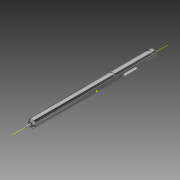
# Autodesk Inventor part: Motor shaft
Saved by Autodesk Inventor 2015 (Build 190141000, 141)
## iProperties
Created: 2008-06-08
Part Number: Motor shaft
Document SubType Name: Modeling
Designer: tangg
Density: 7.84 g/cm^3
Mass: 17.005 g
Surface Area: 63.6795 cm^2
Volume: 17.005 cm^3
Material: Steel, High Strength Low Alloy
Appearance: Steel - Polished
Author: tangg
Autodesk Inventor part; units mm, degrees
ref_plane "XZ Plane" through (0, 0, 0) normal (0, 1, 0) x (-1, 0, 0)
sketch "Sketch1" plane through (0, 0, 0) normal (0, 0, 1) x (1, 0, 0)
  circle A0 centre (0, 0) radius 5
  dimension "d0" = 10
  constraints: 1 centre point, 1 coincident
  measures "d0" diameter of A0
extrude "Extrusion1" add sketch "Sketch1" along normal mid plane 152.4
ref_plane "Work Plane4" through (0, 0, 0) normal (0, 0, 1) x (1, 0, 0)
ref_plane "Work Plane5" through (0, 0, -2) normal (0, 0, 1) x (1, 0, 0)
ref_plane "Work Plane6" through (5, 0, 0) normal (1, 0, 0) x (0, 1, 0)
sketch "Sketch6" plane through (5, 0, 0) normal (1, 0, 0) x (0, 1, 0)
  point P0 (0, 0)
sketch "Sketch7" plane through (5, 0, 0) normal (1, 0, 0) x (0, 1, 0)
  line L0 (0, 106.68) -> (0, -106.68) projected
  line L1 (-1.5, -49.2154) -> (-1.5272, -34.9251)
  line L2 (1.4728, -34.9193) -> (1.5, -49.2096)
  arc A0 (-1.5, -49.2154) -> (1.5, -49.2096) centre (0, -49.2125) ccw
  arc A1 (1.4728, -34.9193) -> (-1.5272, -34.9251) centre (-0.0272, -34.9222) ccw
  line L3 (-1.5, -49.2154) -> (1.5, -49.2096) construction
  line L4 (-1.5272, -34.9251) -> (1.4728, -34.9193) construction
  point P0 (0, 0)
  dimension "d28" = 3
  constraints: 8 end point, 5 point on circle, 3 tangent, 2 centre point, 2 midpoint, 1 coincident, 1 point on line
  measures "d28" distance between parallel lines of L1 L2
extrude "Extrusion2" cut sketch "Sketch7" against normal blind 3
chamfer "Chamfer2" distance 2 angle 45 1 edges at (-5, 0, -76.2)
chamfer "Chamfer3" distance 2 angle 45 1 edges at (-5, 0, 76.2)
sketch "Sketch8" plane through (0, 0, 76.2) normal (0, 0, 1) x (1, 0, 0)
  circle A0 centre (0, 0) radius 1
  dimension "d48" = 2
  constraints: 1 centre point, 1 coincident
  measures "d48" diameter of A0
extrude "Extrusion3" add sketch "Sketch8" along normal blind 6
fillet "Fillet1" radius 0.2 1 edges at (-1, 0, 82.2)
sketch "Sketch9" plane through (0, 0, 0) normal (1, 0, 0) x (0, 1, 0)
  line L0 (-5, -74.2) -> (5, -74.2) projected
  line L1 (-1.5, -49.2154) -> (-1.5272, -34.9251) projected
  line L2 (1.4728, -34.9193) -> (1.5, -49.2096) projected
  line L3 (5, 74.2) -> (-5, 74.2) projected
  line L4 (-5, -74.2) -> (-5, 74.2) projected
  circle A0 centre (-5, -69.85) radius 1
  circle A1 centre (-5, -23.8125) radius 0.75
  line L5 (0, -103.88) -> (0, 103.88) projected
  point P0 (0, 0)
  point P1 (0, -50.7125)
  point P2 (0, -33.4224)
  dimension "d53" = 2
  dimension "d54" = 1.5
  constraints: 2 centre point, 2 point on line, 4 other
  measures "d53" diameter of A0
  measures "d54" diameter of A1
revolve "Revolution4" cut sketch "Sketch9" angle 360 about axis through (0, 0, -10) along (0, 0, 1) contours A0 L4 | L4 A0 | A1 L4 | L4 A1
body "Solid1"
